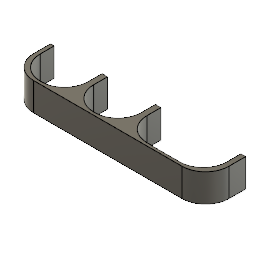
spacer v5 (Autodesk Fusion 360 design; units mm, degrees)
Autodesk Fusion 360 part; units mm, degrees
sketch "Sketch1" plane through (0, 0, 0) normal (0, 0, 1) x (1, 0, 0)
  line L0 (12.555, -6) -> (10.175, -6)
  line L1 (10.175, -6) -> (10.175, 6)
  line L2 (10.175, 6) -> (12.555, 6)
  line L3 (12.555, 6) -> (12.555, -6)
  line L4 (-10.175, -6) -> (-11.775, -6)
  line L5 (-11.775, -6) -> (-11.775, 6)
  line L6 (-11.775, 6) -> (-10.175, 6)
  line L7 (-10.175, 6) -> (-10.175, -6)
  line L8 (0, 0) -> (0, 40) construction
  line L9 (0, 0) -> (20.35, 0) construction
  line L10 (10.175, 6) -> (-10.175, 6)
  line L11 (-10.175, -6) -> (10.175, -6)
  line L12 (12.555, -6) -> (32.905, -6)
  line L13 (32.905, -6) -> (32.905, 6)
  line L14 (32.905, 6) -> (12.555, 6)
  line L15 (12.555, 6) -> (12.555, -6)
  line L16 (32.905, 6) -> (35.285, 6)
  line L17 (35.285, 6) -> (35.285, -6)
  line L18 (35.285, -6) -> (32.905, -6)
  line L19 (32.905, -6) -> (32.905, 6)
  line L20 (35.285, 6) -> (69.285, 6)
  line L21 (69.285, 6) -> (69.285, -6)
  line L22 (69.285, -6) -> (35.285, -6)
  line L23 (35.285, -6) -> (35.285, 6)
  line L24 (69.285, 6) -> (71.385, 6)
  line L25 (71.385, 6) -> (71.385, -6)
  line L26 (71.385, -6) -> (69.285, -6)
  line L27 (69.285, -6) -> (69.285, 6)
  dimension "d1" = 12
  dimension "d2" = 12
  dimension "d3" = 1.6
  dimension "d4" = 2.38
  dimension "d5" = 20.35
  dimension "d12" = 20.35
  dimension "d13" = 2.38
  dimension "d14" = 34
  dimension "d15" = 2.1
extrude "Extrude1" add sketch "Sketch1" along normal blind 16 contours L0 L1 L2 L3 L15 | L13 L16 L17 L18 L19 L23 | L4 L5 L6 L7 | L21 L24 L25 L26 L27 makes body 1 at (10.175, -2, 5.3333) makes body 2 at (-10.175, 2, 5.3333) makes body 3 at (35.285, 2, 5.3333) makes body 4 at (69.285, 2, 5.3333)
extrude "Extrude2" add sketch "Sketch1" along normal blind 1.2 from surface at 16 bodies 2 3 1 4
fillet "Fillet1" radius 10 8 edges at (71.385, 0, 17.2) (-11.775, 0, 17.2) (-10.175, 0, 16) (10.175, 0, 16) (12.555, 0, 16) (32.905, 0, 16) (35.285, 0, 16) (69.285, 0, 16) on bodies 2
equation "d1 = d2"
equation "d12 = d5"
